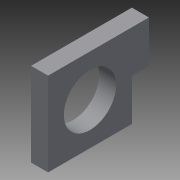
# Autodesk Inventor part: body-side2
Saved by Autodesk Inventor 2013 (Build 170138000, 138)
## iProperties
Created: 2012-09-08
Part Number: body-side2
Material: Generic
Document SubType Name: Modeling
Designer: frankenteddy
Density: 1 g/cm^3
Author: frankenteddy
Autodesk Inventor part; units mm, degrees
ref_plane "YZ Plane" through (0, 0, 0) normal (1, 0, 0) x (0, 1, 0)
ref_plane "XZ Plane" through (0, 0, 0) normal (0, 1, 0) x (-1, 0, 0)
ref_plane "XY Plane" through (0, 0, 0) normal (0, 0, 1) x (1, 0, 0)
sketch "Sketch1" plane through (0, 0, 0) normal (1, 0, 0) x (0, 1, 0)
  line L0 (-92.7646, -8.503) -> (-89.7646, -8.503)
  line L1 (-89.7646, -8.503) -> (-89.7646, -11.753)
  line L2 (-89.7646, -11.753) -> (-92.7646, -11.753)
  line L3 (-92.7646, -11.753) -> (-92.7646, -8.503)
  line L4 (-92.7646, -21.6527) -> (-89.7646, -21.6527)
  line L5 (-89.7646, -21.6527) -> (-89.7646, -21.7527)
  line L6 (-89.7646, -21.7527) -> (-92.7646, -21.7527)
  line L7 (-92.7646, -21.7527) -> (-92.7646, -21.6527)
  circle A0 centre (0, 0) radius 5
  line L8 (-8, -8) -> (8, -8)
  line L9 (8, -8) -> (8, 8)
  line L10 (8, 8) -> (-8, 8)
  line L11 (-8, 8) -> (-8, -8)
  line L12 (-8, 0) -> (8, 0) construction
  line L13 (0, 8) -> (0, -8) construction
  line L14 (8, 8) -> (11.25, 8)
  line L15 (11.25, 8) -> (11.25, 0)
  line L16 (11.25, 0) -> (8, 0)
  line L17 (8, 0) -> (8, 8)
  dimension "d0" = 3
  dimension "mat" = 3.25
  dimension "d2" = 3
  dimension "kerf" = 0.1
  dimension "d22" = 10
  dimension "d23" = 16
  dimension "d24" = 16
  dimension "d25" = 3.25
  dimension "d26" = 8
  constraints: 36 end point, 8 midpoint, 8 parallel, 4 horizontal, 4 perpendicular, 1 centre point
  measures "d0" distance of L1.end L2.end
  measures "mat" distance of L0.end L1.end
  measures "d2" distance of L5.end L6.end
  measures "kerf" distance of L4.end L5.end
  measures "d22" diameter of A0
  measures "d23" distance of L10.end L9.end
  measures "d24" distance of L9.end L8.end
  measures "d25" distance of L15.end L16.end
  measures "d26" distance of L14.end L15.end
extrude "Extrusion3" add sketch "Sketch1" along normal blind 3.25 contours L11 L10 L9 L8 | L9 L14 L15 L16
equation "\"d25\" = mat"
equation "\"d27\" = mat"
body "Solid2"
